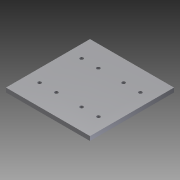
# Autodesk Inventor part: union
Saved by Autodesk Inventor 2011 (Build 150239000, 239)
## iProperties
Created: 2010-08-08
Part Number: union
Document SubType Name: Modeling
Designer: lucio
Density: 1 g/cm^3
Author: lucio
Autodesk Inventor part; units mm, degrees
ref_plane "YZ Plane" through (0, 0, 0) normal (1, 0, 0) x (0, 1, 0)
ref_plane "XZ Plane" through (0, 0, 0) normal (0, 1, 0) x (-1, 0, 0)
ref_plane "XY Plane" through (0, 0, 0) normal (0, 0, 1) x (1, 0, 0)
sketch "Sketch1" plane through (0, 0, 0) normal (0, 0, 1) x (1, 0, 0)
  line L0 (-21.3772, 10.6587) -> (78.6228, 10.6587)
  line L1 (78.6228, 10.6587) -> (78.6228, -89.3413)
  line L2 (78.6228, -89.3413) -> (-21.3772, -89.3413)
  line L3 (-21.3772, -89.3413) -> (-21.3772, 10.6587)
  point P0 (0, 0)
  dimension "d0" = 100
  dimension "d1" = 100
  constraints: 8 end point, 2 parallel, 1 horizontal, 1 perpendicular
  measures "d0" distance of L0.start L0.end
  measures "d1" distance of L2.end L0.start
extrude "Extrusion1" add sketch "Sketch1" along normal blind 5
sketch "Sketch2" plane through (0, 0, 5) normal (0, 0, 1) x (1, 0, 0)
  line L0 (78.6228, 10.6587) -> (78.6228, -89.3413) projected
  line L1 (-21.3772, 10.6587) -> (78.6228, 10.6587) projected
  line L2 (-21.3772, -89.3413) -> (-21.3772, 10.6587) projected
  line L3 (78.6228, -89.3413) -> (-21.3772, -89.3413) projected
  point P0 (0, 0)
  point P1 (-6.3772, -64.3413)
  point P2 (-6.3772, -14.3413)
  point P3 (13.6228, -64.3413)
  point P4 (13.6228, -14.3413)
  point P5 (43.6228, -64.3413)
  point P6 (43.6228, -14.3413)
  point P7 (63.6228, -14.3413)
  point P8 (63.6228, -64.3413)
  dimension "d4" = 25
  dimension "d5" = 25
  dimension "d6" = 15
  dimension "d7" = 20
  dimension "d8" = 15
  dimension "d9" = 20
  constraints: 6 horizontal alignment, 4 vertical alignment
  measures "d4" distance from line of L1 point (-6.377, -14.341)
  measures "d5" distance from line of L3 point (-6.377, -64.341)
  measures "d6" distance from line of L2 point (-6.377, -14.341)
  measures "d7" distance of point (13.623, -14.341) point (-6.377, -14.341)
  measures "d8" distance from line of L0 point (63.623, -14.341)
  measures "d9" distance of point (43.623, -14.341) point (63.623, -14.341)
hole "Hole1" at (-6.3772, -64.3413, 5) at (-6.3772, -14.3413, 5) at (13.6228, -64.3413, 5) at (13.6228, -14.3413, 5) at (43.6228, -64.3413, 5) at (43.6228, -14.3413, 5) at (63.6228, -14.3413, 5) at (63.6228, -64.3413, 5) direction (0, 0, -1) diameter 4 end through all
body "Solid1"
